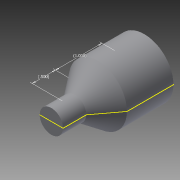
# Autodesk Inventor part: motor connector
Saved by Autodesk Inventor 2014 SP1 (Build 180222100, 222)
## iProperties
Created: 2014-02-07
Part Number: motor connector
Material: Generic
Document SubType Name: Modeling
Designer: Owner
Density: 1 g/cm^3
Appearance: Default
Author: Owner
Autodesk Inventor part; units mm, degrees
ref_plane "YZ Plane" through (0, 0, 0) normal (1, 0, 0) x (0, 1, 0)
ref_plane "XZ Plane" through (0, 0, 0) normal (0, 1, 0) x (-1, 0, 0)
ref_plane "XY Plane" through (0, 0, 0) normal (0, 0, 1) x (1, 0, 0)
sketch "Sketch1" plane through (0, 0, 0) normal (0, 0, 1) x (1, 0, 0)
  circle A0 centre (0, 0) radius 15.875
  arc A1 (-3.0359, 9.528) -> (-6.5275, 7.5757) centre (0, 0) ccw
  line L0 (0, 0) -> (-5, 8.6603) construction
  line L1 (0, 0) -> (-10.16, 0) construction
  line L2 (-2.058, 7.8342) -> (-3.0359, 9.528)
  line L3 (-5.5564, 5.8937) -> (-6.5275, 7.5757)
  arc A2 (-2.058, 7.8342) -> (-5.5564, 5.8937) centre (0, 0) ccw
  circle A3 centre (0, 0) radius 8.1
  arc A4 (6.7336, 7.3932) -> (3.297, 9.4409) centre (0, 0) ccw
  line L4 (5.7556, 5.6994) -> (6.7336, 7.3932)
  line L5 (2.3259, 7.7589) -> (3.297, 9.4409)
  arc A5 (9.7695, -2.1348) -> (9.8245, 1.8652) centre (0, 0) ccw
  line L6 (7.8136, -2.1348) -> (9.7695, -2.1348)
  line L7 (7.8823, 1.8652) -> (9.8245, 1.8652)
  arc A6 (3.0359, -9.528) -> (6.5275, -7.5757) centre (0, 0) ccw
  line L8 (2.058, -7.8342) -> (3.0359, -9.528)
  line L9 (5.5564, -5.8937) -> (6.5275, -7.5757)
  arc A7 (-6.7336, -7.3932) -> (-3.297, -9.4409) centre (0, 0) ccw
  line L10 (-5.7556, -5.6994) -> (-6.7336, -7.3932)
  line L11 (-2.3259, -7.7589) -> (-3.297, -9.4409)
  arc A8 (-9.7695, 2.1348) -> (-9.8245, -1.8652) centre (0, 0) ccw
  line L12 (-7.8136, 2.1348) -> (-9.7695, 2.1348)
  line L13 (-7.8823, -1.8652) -> (-9.8245, -1.8652)
  point P0 (5, 8.6603)
  point P1 (10, 0)
  point P2 (5, -8.6603)
  point P3 (-5, -8.6603)
  point P4 (-10, 0)
  dimension "d5" = 16.2
  dimension "d0" = 31.75
  dimension "d2" = 60
  dimension "d3" = 4
  dimension "d4" = 20
  dimension "d8" = 360
  constraints: 34 end point, 20 point on circle, 8 centre point, 5 coincident, 2 parallel, 1 horizontal, 61 other
  measures "d0" diameter of A0
  measures "d2" angle of L1 L0
  measures "d3" distance between parallel lines of L2 L3
  measures "d4" diameter of A1
extrude "Extrusion1" add sketch "Sketch1" along normal blind 25.4 contours A0 | L2 A2 L3 A1 | A3 A2 | L5 A4 L4 A3 | A3 L13 A8 L12 | L7 A5 L6 A3 | A3 L11 A7 L10 | A3 L9 A6 L8
extrude "Extrusion2" cut sketch "Sketch1" along normal blind 15.24 contours A3 A2
extrude "Extrusion3" cut sketch "Sketch1" along normal blind 15.24 contours L2 A2 L3 A1
pattern_circular "Circular Pattern1" count 6 over 360 about axis through (0, 0, 0) along (0, 0, 1) of "Extrusion3"
sketch "Sketch2" plane through (0, 0, 15.24) normal (0, 0, -1) x (-1, 0, 0)
  arc A0 (9.8245, -1.8652) -> (9.7695, 2.1348) centre (0, 0) ccw projected
  circle A1 centre (0, 0) radius 4.7625
  dimension "d19" = 9.525
  constraints: 1 centre point, 1 coincident
  measures "d19" diameter of A1
extrude "Extrusion4" cut sketch "Sketch2" against normal blind 7.62
sketch "Sketch4" plane through (0, 0, 0) normal (1, 0, 0) x (0, 1, 0)
  line L0 (8.1, 0) -> (8.1, 15.24) projected
  line L1 (8.1, 15.24) -> (4.7625, 15.24) projected
  line L2 (4.7625, 15.24) -> (4.7625, 22.86) projected
  line L3 (4.7625, 22.86) -> (-4.7625, 22.86) projected
  line L4 (-4.7625, 22.86) -> (-4.7625, 15.24) projected
  line L5 (-4.7625, 15.24) -> (-8.1, 15.24) projected
  line L6 (-8.1, 15.24) -> (-8.1, 0) projected
  line L7 (-8.1, 0) -> (-15.875, 0) projected
  line L8 (-15.875, 0) -> (-15.875, 25.4) projected
  line L9 (-15.875, 25.4) -> (15.875, 25.4) projected
  line L10 (15.875, 25.4) -> (15.875, 0) projected
  line L11 (15.875, 0) -> (8.1, 0) projected
  line L12 (0, 25.4) -> (0, 50.8)
  line L13 (0, 50.8) -> (-6.35, 50.8)
  line L14 (-6.35, 50.8) -> (-6.35, 38.1)
  line L15 (-6.35, 38.1) -> (-15.875, 25.4)
  point P0 (0, 0)
  dimension "d22" = 25.4
  dimension "d23" = 6.35
  dimension "d24" = 12.7
  constraints: 8 end point, 2 perpendicular, 1 midpoint, 1 parallel
  measures "d22" distance of L12.start L12.end
  measures "d23" distance of L12.end L13.end
  measures "d24" distance of L13.end L14.end
revolve "Revolution1" add sketch "Sketch4" angle 360 about axis through (0, 0, 25.4) along (0, 0, 1) contours L9 L15 L14 L13 L12
sketch "Sketch5" plane through (0, 0, 0) normal (0, 1, 0) x (-1, 0, 0)
  line L0 (10, 0) -> (10, 15.24) projected
  line L1 (10, 15.24) -> (4.7625, 15.24) projected
  line L2 (4.7625, 15.24) -> (4.7625, 22.86) projected
  line L3 (4.7625, 22.86) -> (-4.7625, 22.86) projected
  line L4 (-4.7625, 22.86) -> (-4.7625, 15.24) projected
  line L5 (-4.7625, 15.24) -> (-10, 15.24) projected
  line L6 (-10, 15.24) -> (-10, 0) projected
  line L7 (-10, 0) -> (-15.875, 0) projected
  line L8 (-15.875, 0) -> (-15.875, 25.4) projected
  line L9 (-15.875, 25.4) -> (-6.35, 38.1) projected
  line L10 (-6.35, 38.1) -> (-6.35, 50.8) projected
  line L11 (-6.35, 50.8) -> (6.35, 50.8) projected
  line L12 (6.35, 50.8) -> (6.35, 38.1) projected
  line L13 (6.35, 38.1) -> (15.875, 25.4) projected
  line L14 (15.875, 25.4) -> (15.875, 0) projected
  line L15 (15.875, 0) -> (10, 0) projected
  point P0 (0, 0)
  dimension "d26" = 25.4
  dimension "d27" = 12.7
  measures "d26" distance of L13.end L14.end
  measures "d27" vertical distance of L12.end L13.end
body "Solid1"
